Autodesk Inventor part; units mm, degrees
(part 2 of 2)
  line L98 (-1.068678, -16.78389) -> (-1.338835, -19.958356)
  line L99 (3.754408, -16.652552) -> (3.155195, -19.752961)
  line L100 (3.827782, -16.947395) -> (3.754408, -16.652552)
  line L101 (4.564116, -16.764153) -> (3.827782, -16.947395)
  line L102 (4.429221, -16.222095) -> (4.564116, -16.764153)
  line L103 (3.692887, -16.405337) -> (4.429221, -16.222095)
  line L104 (3.738969, -16.590512) -> (3.692887, -16.405337)
  line L105 (3.001118, -16.694525) -> (3.738969, -16.590512)
  line L106 (2.633978, -18.835494) -> (3.001118, -16.694525)
  line L107 (1.686844, -16.879795) -> (2.633978, -18.835494)
  line L108 (0.901216, -16.990543) -> (1.686844, -16.879795)
  line L109 (1.257518, -17.690231) -> (0.901216, -16.990543)
  line L110 (0.599517, -17.695015) -> (1.257518, -17.690231)
  line L111 (0.157714, -19.141701) -> (0.599517, -17.695015)
  line L112 (-0.337209, -17.701826) -> (0.157714, -19.141701)
  line L113 (-1.088567, -17.707289) -> (-0.337209, -17.701826)
  line L114 (-0.229443, -19.945348) -> (-1.088567, -17.707289)
  line L115 (-0.571394, -20.847534) -> (-0.229443, -19.945348)
  line L116 (0.199736, -20.841927) -> (-0.571394, -20.847534)
  line L117 (1.303377, -17.780286) -> (0.199736, -20.841927)
  line L118 (2.364672, -19.864399) -> (1.303377, -17.780286)
  line L119 (3.155195, -19.752961) -> (2.364672, -19.864399)
  line L120 (5.177609, -19.321511) -> (4.482049, -19.494606)
  line L121 (4.482049, -19.494606) -> (3.926354, -17.261618)
  line L122 (3.926354, -17.261618) -> (4.621915, -17.088523)
  line L123 (4.621915, -17.088523) -> (5.177609, -19.321511)
  spline S89 degree 2 poles (6.390481, -19.017051) (6.15193, -19.098607) (5.687961, -19.139683) (5.52365, -19.117495) knots 0 0 0 0.5 1 1 1
  line L124 (5.52365, -19.117495) -> (5.327757, -18.544504)
  line L125 (5.327757, -18.544504) -> (5.383887, -18.525314)
  spline S90 degree 2 poles (5.383887, -18.525314) (5.445793, -18.545943) (5.60013, -18.592439) (5.726841, -18.603973) knots 0 0 0 0.5 1 1 1
  spline S91 degree 2 poles (5.726841, -18.603973) (5.837921, -18.615627) (6.095722, -18.598017) (6.236046, -18.550044) knots 0 0 0 0.5 1 1 1
  spline S92 degree 2 poles (6.236046, -18.550044) (6.378709, -18.50127) (6.568167, -18.33724) (6.535385, -18.241351) knots 0 0 0 0.5 1 1 1
  spline S93 degree 2 poles (6.535385, -18.241351) (6.509799, -18.166512) (6.382048, -18.121376) (6.225853, -18.138206) knots 0 0 0 0.5 1 1 1
  spline S94 degree 2 poles (6.225853, -18.138206) (6.141478, -18.143543) (5.890074, -18.179863) (5.789269, -18.182981) knots 0 0 0 0.5 1 1 1
  spline S95 degree 2 poles (5.789269, -18.182981) (5.504822, -18.191415) (5.14122, -17.968315) (5.054068, -17.713393) knots 0 0 0 0.5 1 1 1
  spline S96 degree 2 poles (5.054068, -17.713393) (5.004495, -17.568391) (5.049851, -17.265555) (5.146439, -17.120214) knots 0 0 0 0.5 1 1 1
  spline S97 degree 2 poles (5.146439, -17.120214) (5.241488, -16.978011) (5.582725, -16.730746) (5.823614, -16.648391) knots 0 0 0 0.5 1 1 1
  spline S98 degree 2 poles (5.823614, -16.648391) (6.052811, -16.570034) (6.467547, -16.530117) (6.620104, -16.548487) knots 0 0 0 0.5 1 1 1
  line L126 (6.620104, -16.548487) -> (6.8088, -17.100429)
  line L127 (6.8088, -17.100429) -> (6.755009, -17.118819)
  spline S99 degree 2 poles (6.755009, -17.118819) (6.710334, -17.102748) (6.527133, -17.063508) (6.445777, -17.054753) knots 0 0 0 0.5 1 1 1
  spline S100 degree 2 poles (6.445777, -17.054753) (6.346451, -17.046917) (6.118374, -17.067425) (6.008453, -17.105004) knots 0 0 0 0.5 1 1 1
  spline S101 degree 2 poles (6.008453, -17.105004) (5.861113, -17.155377) (5.692024, -17.325504) (5.720008, -17.40736) knots 0 0 0 0.5 1 1 1
  spline S102 degree 2 poles (5.720008, -17.40736) (5.745594, -17.4822) (5.874944, -17.532013) (6.057725, -17.516542) knots 0 0 0 0.5 1 1 1
  spline S103 degree 2 poles (6.057725, -17.516542) (6.151455, -17.508007) (6.391905, -17.470208) (6.509141, -17.469309) knots 0 0 0 0.5 1 1 1
  spline S104 degree 2 poles (6.509141, -17.469309) (6.768601, -17.464192) (7.111775, -17.67338) (7.194929, -17.916609) knots 0 0 0 0.5 1 1 1
  spline S105 degree 2 poles (7.194929, -17.916609) (7.246901, -18.068627) (7.199385, -18.39571) (7.09806, -18.534834) knots 0 0 0 0.5 1 1 1
  spline S106 degree 2 poles (7.09806, -18.534834) (6.995255, -18.684913) (6.654758, -18.926701) (6.390481, -19.017051) knots 0 0 0 0.5 1 1 1
  line L128 (19.259047, 5.629037) -> (19.447781, 4.716544)
  line L129 (18.196092, 4.361742) -> (19.259047, 5.629037)
  line L130 (19.447781, 4.716544) -> (18.523051, 3.659563)
  spline S107 degree 2 poles (17.182895, 4.745308) (17.524173, 4.815895) (18.016664, 4.594693) (18.196092, 4.361742) knots 0 0 0 0.5 1 1 1
  line L131 (18.523051, 3.659563) -> (18.57912, 3.388478)
  spline S108 degree 2 poles (16.594214, 4.260099) (16.66283, 4.440872) (16.940855, 4.695246) (17.182895, 4.745308) knots 0 0 0 0.5 1 1 1
  line L132 (18.57912, 3.388478) -> (19.675564, 3.615259)
  spline S109 degree 2 poles (16.594666, 3.452528) (16.543102, 3.70183) (16.529938, 4.082748) (16.594214, 4.260099) knots 0 0 0 0.5 1 1 1
  line L133 (19.675564, 3.615259) -> (19.829756, 2.869774)
  line L134 (16.842974, 2.252007) -> (16.594666, 3.452528)
  line L135 (19.829756, 2.869774) -> (16.842974, 2.252007)
  spline S110 degree 2 poles (17.804882, 3.922426) (17.731774, 3.983023) (17.56235, 4.021175) (17.436489, 3.995143) knots 0 0 0 0.5 1 1 1
  spline S111 degree 2 poles (17.436489, 3.995143) (17.32273, 3.971614) (17.178585, 3.850937) (17.155543, 3.742689) knots 0 0 0 0.5 1 1 1
  spline S112 degree 2 poles (17.155543, 3.742689) (17.141016, 3.66649) (17.159617, 3.491137) (17.18615, 3.362855) knots 0 0 0 0.5 1 1 1
  line L136 (17.18615, 3.362855) -> (17.238215, 3.111133)
  line L137 (17.238215, 3.111133) -> (18.04179, 3.27734)
  line L138 (18.04179, 3.27734) -> (17.997235, 3.492756)
  spline S113 degree 2 poles (17.997235, 3.492756) (17.965195, 3.647662) (17.880912, 3.859909) (17.804882, 3.922426) knots 0 0 0 0.5 1 1 1
  spline S114 degree 2 poles (18.829313, 6.926439) (19.048234, 6.311747) (18.694503, 5.448503) (18.151991, 5.255288) knots 0 0 0 0.5 1 1 1
  spline S115 degree 2 poles (18.584841, 7.413963) (18.654084, 7.31531) (18.769607, 7.094082) (18.829313, 6.926439) knots 0 0 0 0.5 1 1 1
  spline S116 degree 2 poles (18.151991, 5.255288) (17.621121, 5.066219) (16.77054, 5.450697) (16.574837, 6.000194) knots 0 0 0 0.5 1 1 1
  spline S117 degree 2 poles (18.347351, 7.712444) (18.409802, 7.640232) (18.513779, 7.525088) (18.584841, 7.413963) knots 0 0 0 0.5 1 1 1
  spline S118 degree 2 poles (16.574837, 6.000194) (16.398207, 6.496138) (16.756944, 7.190624) (17.255216, 7.368083) knots 0 0 0 0.5 1 1 1
  line L139 (17.788541, 7.513424) -> (18.347351, 7.712444)
  line L140 (17.255216, 7.368083) -> (17.499696, 7.455155)
  line L141 (17.814248, 7.441244) -> (17.788541, 7.513424)
  line L142 (17.499696, 7.455155) -> (18.027928, 5.971979)
  spline S119 degree 2 poles (18.063284, 7.228211) (17.998506, 7.299594) (17.862601, 7.408614) (17.814248, 7.441244) knots 0 0 0 0.5 1 1 1
  spline S120 degree 2 poles (18.027928, 5.971979) (18.175955, 6.035194) (18.337221, 6.215943) (18.366247, 6.325982) knots 0 0 0 0.5 1 1 1
  spline S121 degree 2 poles (18.315476, 6.822147) (18.274014, 6.938566) (18.141523, 7.148504) (18.063284, 7.228211) knots 0 0 0 0.5 1 1 1
  spline S122 degree 2 poles (18.366247, 6.325982) (18.396102, 6.433692) (18.364402, 6.684773) (18.315476, 6.822147) knots 0 0 0 0.5 1 1 1
  line L143 (17.621291, 5.824532) -> (17.329395, 6.64412)
  spline S123 degree 2 poles (17.329395, 6.64412) (17.116843, 6.563173) (16.95816, 6.294137) (17.026988, 6.100882) knots 0 0 0 0.5 1 1 1
  spline S124 degree 2 poles (17.026988, 6.100882) (17.097474, 5.90297) (17.414576, 5.764029) (17.621291, 5.824532) knots 0 0 0 0.5 1 1 1
  line L144 (15.275905, 9.020575) -> (17.702871, 9.314447)
  line L145 (17.702871, 9.314447) -> (18.054181, 8.614113)
  line L146 (18.054181, 8.614113) -> (16.364188, 6.851086)
  line L147 (16.364188, 6.851086) -> (16.026178, 7.524909)
  line L148 (16.026178, 7.524909) -> (17.173198, 8.628439)
  line L149 (17.173198, 8.628439) -> (15.607266, 8.360007)
  line L150 (15.607266, 8.360007) -> (15.275905, 9.020575)
  line L151 (15.221292, 13.018303) -> (16.446221, 11.41915)
  line L152 (16.446221, 11.41915) -> (16.024359, 11.096009)
  line L153 (16.024359, 11.096009) -> (15.633584, 11.606169)
  line L154 (15.633584, 11.606169) -> (14.352299, 10.624722)
  line L155 (14.352299, 10.624722) -> (14.743074, 10.114563)
  line L156 (14.743074, 10.114563) -> (14.348682, 9.812464)
  spline S125 degree 2 poles (14.348682, 9.812464) (14.263012, 9.924306) (14.063743, 10.123485) (13.981247, 10.16615) knots 0 0 0 0.5 1 1 1
  spline S126 degree 2 poles (13.981247, 10.16615) (13.883388, 10.212614) (13.685792, 10.198249) (13.581673, 10.130949) knots 0 0 0 0.5 1 1 1
  line L157 (13.581673, 10.130949) -> (13.175868, 10.66073)
  line L158 (13.175868, 10.66073) -> (15.181187, 12.196776)
  line L159 (15.181187, 12.196776) -> (14.79943, 12.695163)
  line L160 (14.79943, 12.695163) -> (15.221292, 13.018303)
  line L161 (14.344815, 13.94118) -> (14.840085, 13.412826)
  line L162 (14.840085, 13.412826) -> (14.252223, 12.861775)
  line L163 (14.252223, 12.861775) -> (13.756953, 13.390129)
  line L164 (13.756953, 13.390129) -> (14.344815, 13.94118)
  spline S127 degree 2 poles (11.273228, 14.684046) (11.533476, 14.981806) (12.018758, 15.345493) (12.256586, 15.40352) knots 0 0 0 0.5 1 1 1
  spline S128 degree 2 poles (10.699744, 13.626029) (10.727278, 13.867857) (11.021113, 14.395591) (11.273228, 14.684046) knots 0 0 0 0.5 1 1 1
  spline S129 degree 2 poles (12.256586, 15.40352) (12.490926, 15.461314) (12.961144, 15.319511) (13.203075, 15.108059) knots 0 0 0 0.5 1 1 1
  spline S130 degree 2 poles (11.112959, 12.716672) (10.865446, 12.933003) (10.670818, 13.378853) (10.699744, 13.626029) knots 0 0 0 0.5 1 1 1
  spline S131 degree 2 poles (13.203075, 15.108059) (13.446866, 14.894981) (13.648469, 14.4496) (13.621169, 14.204285) knots 0 0 0 0.5 1 1 1
  spline S132 degree 2 poles (12.059448, 12.421211) (11.818133, 12.362948) (11.347445, 12.511727) (11.112959, 12.716672) knots 0 0 0 0.5 1 1 1
  spline S133 degree 2 poles (13.621169, 14.204285) (13.595496, 13.96083) (13.303288, 13.434958) (13.04304, 13.137198) knots 0 0 0 0.5 1 1 1
  spline S134 degree 2 poles (13.04304, 13.137198) (12.776286, 12.831993) (12.304016, 12.483195) (12.059448, 12.421211) knots 0 0 0 0.5 1 1 1
  spline S135 degree 2 poles (12.832221, 14.683751) (12.668453, 14.826887) (12.221226, 14.600637) (11.851999, 14.178189) knots 0 0 0 0.5 1 1 1
  spline S136 degree 2 poles (11.851999, 14.178189) (11.47952, 13.75202) (11.318183, 13.285743) (11.483812, 13.14098) knots 0 0 0 0.5 1 1 1
  spline S137 degree 2 poles (11.483812, 13.14098) (11.649441, 12.996218) (12.091789, 13.216885) (12.465895, 13.644916) knots 0 0 0 0.5 1 1 1
  spline S138 degree 2 poles (12.465895, 13.644916) (12.833495, 14.065502) (12.997851, 14.538988) (12.832221, 14.683751) knots 0 0 0 0.5 1 1 1
extrude "Wyciągnięcie proste2" add sketch "Szkic3 outline for Wyciągnięcie proste2" along normal blind 0.3
equation "\"d13\" = name_plate_d"
equation "\"d14\" = name_plate_D"
equation "\"d15\" = name_plate_insert_r"
equation "\"d6\" = insert_m2_pocket_d"
equation "\"d8\" = insert_m2_pocket_D"
equation "\"d9\" = insert_m2_pocket_nut_h"
equation "\"d16\" = name_plate_text_d"
equation "\"insert_m2_d\" = 2.9"
equation "\"insert_m2_h\" = 7"
equation "\"insert_m2_corner\" = 0.5"
equation "\"insert_m2_pocket_d\" = 2.6"
equation "\"insert_m2_pocket_D\" = 4.5"
equation "\"insert_m2_pocket_nut_h\" = 1.5"
equation "\"stator_r_out\" = 30.15"
equation "\"stator_out_d\" = 3.2"
equation "\"stator_h\" = 45"
equation "\"stator_radial_screw_d\" = 4"
equation "\"stator_radial_screw_pos\" = 4"
equation "\"mag_size_x\" = 7"
equation "\"mag_size_y\" = 3"
equation "\"mag_corner_r\" = 0.4"
equation "\"magnet_ring_r\" = 26.95"
equation "\"magnet_ring_d\" = 3.3"
equation "\"magnet_ring_h\" = 36"
equation "\"magnet_ring_pocket_mag_size_x\" = 7.1"
equation "\"magnet_ring_pocket_mag_size_y\" = 3.1"
equation "\"magnet_ring_pocket_mag_size_z\" = 10.1"
equation "\"magnet_ring_pocket_radial_cut\" = 1.4"
equation "\"magnet_ring_insert_part_lengthen\" = 8"
equation "\"magnet_ring_insert_part_axial_flat_cut\" = 0.17"
equation "\"magnet_ring_insert_pos\" = 4"
equation "\"casing_d\" = 3"
equation "\"casing_r_in\" = 30.15"
equation "\"casing_lock_hole_r\" = 14.25"
equation "\"casing_lock_h\" = 8"
equation "\"casing_stator_fix_r\" = 23"
equation "\"casing_stator_fix_h\" = 6"
equation "\"casing_sidebar_length\" = 3"
equation "\"casing_vent_hole_length\" = 4"
equation "\"casing_vent_hole_width\" = 6"
equation "\"casing_head_insert_r\" = 19"
equation "\"casing_radial_stator_insert_pos\" = 18.1"
equation "\"casing_cart_hole_ang\" = 90deg"
equation "\"casing_cart_hole_width\" = 2.6"
equation "\"casing_cart_hole_corner\" = 1"
equation "\"casing_cart_hole_pos\" = 17"
equation "\"casing_sleeve_cut_d\" = 46"
equation "\"casing_sleeve_cut_h\" = 4"
equation "\"casing_backsleeve_insert_pos\" = 4.9"
equation "\"rotor_out_r\" = 22.5"
equation "\"rotor_coil_groove_in_r\" = 17"
equation "\"rotor_coil_groove_ang\" = 18deg"
equation "\"rotor_core_r\" = 14.97"
equation "\"rotor_coil_groove_in_correction_r\" = 18"
equation "\"rotor_plastic_h\" = 32"
equation "\"rotor_teeth_d\" = 1.5"
equation "\"rotor_plastic_insert_r\" = 37"
equation "\"shaft_d\" = 8"
equation "\"shaft_lock_1_d\" = 8.1"
equation "\"shaft_lock_1_D\" = 44"
equation "\"shaft_lock_1_h1\" = 3.5"
equation "\"shaft_lock_1_corner\" = 2"
equation "\"shaft_lock_1_rotor_insert_grove_d_in\" = 36"
equation "\"shaft_lock_1_rotor_insert_grove_width_out\" = 5.5"
equation "\"shaft_lock_1_rotor_insert_grove_width_in\" = 7.6"
equation "\"shaft_lock_1_rotor_insert_r\" = 37"
equation "\"shaft_lock_1_shaft_insert_axial_cut_out_width\" = 12"
equation "\"shaft_lock_1_shaft_insert_axial_cut_in_width\" = 5.4"
equation "\"shaft_lock_1_shaft_insert_pos\" = 2.5"
equation "\"shaft_lock_1_shaft_insert_corner\" = 2"
equation "\"shaft_lock_1_shaft_insert_corner_finish\" = 0.5"
equation "\"shaft_lock_2_d\" = 8.1"
equation "\"shaft_lock_2_D\" = 44"
equation "\"shaft_lock_2_h1\" = 3.5"
equation "\"shaft_lock_2_corner\" = 2"
equation "\"shaft_lock_2_rotor_insert_grove_d_in\" = 36"
equation "\"shaft_lock_2_rotor_insert_grove_width_out\" = 5.5"
equation "\"shaft_lock_2_rotor_insert_grove_width_in\" = 7.6"
equation "\"shaft_lock_2_rotor_insert_r\" = 37"
equation "\"shaft_lock_2_shaft_insert_axial_cut_out_width\" = 12"
equation "\"shaft_lock_2_shaft_insert_axial_cut_in_width\" = 5.4"
equation "\"shaft_lock_2_shaft_insert_pos\" = 2.5"
equation "\"shaft_lock_2_shaft_insert_corner\" = 2"
equation "\"shaft_lock_2_shaft_insert_corner_finish\" = 0.5"
equation "\"commutator_plastic_shaft_d\" = 8.1"
equation "\"commutator_plastic_h\" = 17"
equation "\"commutator_plastic_insert_cut_deepness\" = 0.5"
equation "\"commutator_plastic_insert_cut_length\" = 6"
equation "\"commutator_plastic_insert_pos\" = 3"
equation "\"commutator_plate_D\" = 22"
equation "\"commutator_plate_d\" = 1"
equation "\"commutator_plate_ang\" = 55deg"
equation "\"commutator_plate_h\" = 17"
equation "\"commutator_plate_insert_pos\" = 3"
equation "\"sleeve_in_r\" = 11.1"
equation "\"sleeve_d\" = 3"
equation "\"sleeve_h\" = 7"
equation "\"sleeve_cup_r\" = 22"
equation "\"sleeve_cup_h\" = 4.5"
equation "\"sleeve_head_insert_r\" = 19"
equation "\"rotor_sleeve_in_D\" = 8.15"
equation "\"rotor_sleeve_out_D\" = 10.5"
equation "\"rotor_sleeve_h\" = 32"
equation "\"carbon_brush_batt_d\" = 4"
equation "\"carbon_brush_batt_h\" = 8"
equation "\"brush_cart_outer_holder_width\" = 5.5"
equation "\"brush_cart_outer_holder_arc_r\" = 33.15"
equation "\"brush_cart_outer_holder_arc_pos\" = 1.5"
equation "\"brush_holder_batt_width\" = 16"
equation "\"brush_holder_batt_arc_r\" = 30.15"
equation "\"brush_holder_batt_insert_flat_length\" = 6"
equation "\"brush_holder_batt_insert_flat_depth\" = 6"
equation "\"brush_holder_batt_brush_hole_d\" = 4.5"
equation "\"name_plate_D\" = 45"
equation "\"name_plate_d\" = 28"
equation "\"name_plate_insert_r\" = 19"
equation "\"name_plate_text_d\" = 40"
equation "\"sleeve_bearing_material_lock_h\" = 2"
equation "\"back_sleeve_D\" = 66"
equation "\"back_sleeve_d\" = 22.2"
equation "\"back_sleeve_h\" = 5"
equation "\"commutator_back_plate_lock_h\" = 2"
equation "\"commutator_back_plate_lock_r\" = 23"
equation "\"commutator_plastic_back_plate_lock_r\" = 11.9"
equation "\"commutator_plastic_back_plate_lock_h\" = 1"
equation "\"commutator_plastic_back_plate_hook_in_r\" = 11.15"
equation "\"commutator_plastic_back_plate_hook_d\" = 1"
